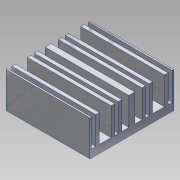
# Autodesk Inventor part: HeatSink
Saved by Autodesk Inventor 2015 (Build 190159000, 159)
## iProperties
Created: 2015-05-21
Part Number: HeatSink
Material: Aluminum 6061
Document SubType Name: Modeling
Designer: Joe Sheldon
Density: 2.7 g/cm^3
Appearance: Aluminum - Flat
Author: Joe Sheldon
Autodesk Inventor part; units mm, degrees
ref_plane "YZ Plane" through (0, 0, 0) normal (1, 0, 0) x (0, 1, 0)
ref_plane "XZ Plane" through (0, 0, 0) normal (0, 1, 0) x (-1, 0, 0)
ref_plane "XY Plane" through (0, 0, 0) normal (0, 0, 1) x (1, 0, 0)
sketch "Sketch1" plane through (0, 0, 0) normal (0, 1, 0) x (-1, 0, 0)
  line L0 (0, 0) -> (-90, 0)
  line L1 (-90, 0) -> (-90, -90)
  line L2 (-90, -90) -> (0, -90)
  line L3 (0, -90) -> (0, 0)
  dimension "d0" = 90
  dimension "d1" = 90
  constraints: 8 end point, 2 parallel, 1 horizontal, 1 perpendicular
  measures "d0" distance of L2.end L1.end
  measures "d1" distance of L1.end L0.end
extrude "Extrusion1" add sketch "Sketch1" along normal blind 88.9
sketch "Sketch2" plane through (90, 0, 0) normal (1, 0, 0) x (0, 0, -1)
  line L0 (0, 0) -> (90, 0) projected
  line L1 (90, 0) -> (90, 88.9) projected
  line L2 (0, 88.9) -> (90, 88.9) projected
  line L3 (0, 0) -> (0, 88.9) projected
  line L4 (0, 88.9) -> (1.6, 88.9)
  line L5 (0, 88.9) -> (90, 88.9) projected
  line L6 (1.6, 88.9) -> (6.2, 88.9)
  line L7 (6.2, 88.9) -> (7.8, 88.9)
  line L8 (7.8, 88.9) -> (7.8, 8.402)
  line L9 (6.2, 88.9) -> (6.2, 8.402)
  line L10 (1.6, 88.9) -> (1.6, 8.402)
  line L11 (1.6, 8.402) -> (6.2, 8.402)
  line L12 (90, 88.9) -> (88.4, 88.9)
  line L13 (88.4, 88.9) -> (88.4, 8.402)
  line L14 (88.4, 8.402) -> (83.8, 8.402)
  line L15 (83.8, 8.402) -> (83.8, 88.9)
  dimension "d4" = 1.6
  dimension "d5" = 4.6
  dimension "d6" = 1.6
  dimension "d7" = 1.6
  dimension "d8" = 4.6
  constraints: 22 end point, 5 perpendicular, 5 point on line, 2 vertical
  measures "d4" distance of L2.start L4.end
  measures "d5" distance of L4.end L6.end
  measures "d6" distance of L6.end L7.end
  measures "d7" distance of L1.end L12.end
  measures "d8" distance of L13.end L14.end
extrude "Extrusion2" cut sketch "Sketch2" against normal blind 127 contours L2 L9 L11 L10 | L13 L14 L15 L2
sketch "Sketch3" plane through (90, 0, 0) normal (1, 0, 0) x (0, 0, -1)
  line L0 (1.6, 8.402) -> (1.6, 88.9) projected
  line L1 (0, 88.9) -> (1.6, 88.9) projected
  line L2 (0, 0) -> (0, 88.9) projected
  line L3 (0, 0) -> (90, 0) projected
  line L4 (90, 0) -> (90, 88.9) projected
  line L5 (88.4, 88.9) -> (90, 88.9) projected
  line L6 (88.4, 88.9) -> (88.4, 8.402) projected
  line L7 (88.4, 8.402) -> (83.8, 8.402) projected
  line L8 (83.8, 8.402) -> (83.8, 88.9) projected
  line L9 (6.2, 88.9) -> (83.8, 88.9) projected
  line L10 (6.2, 88.9) -> (6.2, 8.402) projected
  line L11 (6.2, 8.402) -> (1.6, 8.402) projected
sketch "Sketch5" plane through (90, 0, 0) normal (1, 0, 0) x (0, 0, -1)
  line L0 (-0.0003, 88.9) -> (90, 88.9)
  line L1 (90, 88.9) -> (90, 38.1)
  line L2 (90, 38.1) -> (-0.0003, 38.1)
  line L3 (-0.0003, 38.1) -> (-0.0003, 88.9)
  point P0 (0, 0)
  dimension "d24" = 50.8
  constraints: 8 end point, 2 parallel, 1 horizontal, 1 perpendicular
  measures "d24" distance of L0.end L1.end
extrude "Extrusion3" cut sketch "Sketch5" against normal blind 111.125
sketch "Sketch6" plane through (90, 0, 0) normal (1, 0, 0) x (0, 0, -1)
  line L0 (1.6, 38.1) -> (0, 38.1) projected
  line L1 (0, 0) -> (0, 38.1) projected
  line L2 (0, 0) -> (90, 0) projected
  line L3 (90, 0) -> (90, 38.1) projected
  line L4 (90, 38.1) -> (88.4, 38.1) projected
  line L5 (88.4, 38.1) -> (88.4, 8.402) projected
  line L6 (88.4, 8.402) -> (83.8, 8.402) projected
  line L7 (83.8, 8.402) -> (83.8, 38.1) projected
  line L8 (83.8, 38.1) -> (6.2, 38.1) projected
  line L9 (6.2, 38.1) -> (6.2, 8.402) projected
  line L10 (6.2, 8.402) -> (1.6, 8.402) projected
  line L11 (1.6, 8.402) -> (1.6, 38.1) projected
  line L12 (6.2, 38.1) -> (6.2, 8.402)
  line L13 (6.2, 8.402) -> (10.01, 8.402)
  line L14 (10.01, 8.402) -> (10.01, 38.1)
  line L15 (10.01, 38.1) -> (6.2, 38.1)
  line L16 (10.01, 38.1) -> (10.01, 8.402)
  line L17 (10.01, 8.402) -> (22.71, 8.402)
  line L18 (22.71, 8.402) -> (22.71, 38.1)
  line L19 (22.71, 38.1) -> (10.01, 38.1)
  line L20 (22.71, 38.1) -> (22.71, 8.402)
  line L21 (22.71, 8.402) -> (26.52, 8.402)
  line L22 (26.52, 8.402) -> (26.52, 38.1)
  line L23 (26.52, 38.1) -> (22.71, 38.1)
  line L24 (26.52, 38.1) -> (26.52, 8.402)
  line L25 (26.52, 8.402) -> (30.33, 8.402)
  line L26 (30.33, 8.402) -> (30.33, 38.1)
  line L27 (30.33, 38.1) -> (26.52, 38.1)
  line L28 (30.33, 38.1) -> (30.33, 8.402)
  line L29 (30.33, 8.402) -> (34.14, 8.402)
  line L30 (34.14, 8.402) -> (34.14, 38.1)
  line L31 (34.14, 38.1) -> (30.33, 38.1)
  line L32 (83.8, 38.1) -> (83.8, 8.402)
  line L33 (83.8, 8.402) -> (79.99, 8.402)
  line L34 (79.99, 8.402) -> (79.99, 38.1)
  line L35 (79.99, 38.1) -> (83.8, 38.1)
  line L36 (79.99, 38.1) -> (79.99, 8.402)
  line L37 (79.99, 8.402) -> (67.29, 8.402)
  line L38 (67.29, 8.402) -> (67.29, 38.1)
  line L39 (67.29, 38.1) -> (79.99, 38.1)
  line L40 (67.29, 38.1) -> (67.29, 8.402)
  line L41 (67.29, 8.402) -> (63.48, 8.402)
  line L42 (63.48, 8.402) -> (63.48, 38.1)
  line L43 (63.48, 38.1) -> (67.29, 38.1)
  line L44 (63.48, 38.1) -> (63.48, 8.402)
  line L45 (63.48, 8.402) -> (59.67, 8.402)
  line L46 (59.67, 8.402) -> (59.67, 38.1)
  line L47 (59.67, 38.1) -> (63.48, 38.1)
  line L48 (59.67, 38.1) -> (59.67, 8.402)
  line L49 (59.67, 8.402) -> (55.86, 8.402)
  line L50 (55.86, 8.402) -> (55.86, 38.1)
  line L51 (55.86, 38.1) -> (59.67, 38.1)
  line L52 (55.86, 38.1) -> (55.86, 8.402)
  line L53 (55.86, 8.402) -> (48.24, 8.402)
  line L54 (48.24, 8.402) -> (48.24, 38.1)
  line L55 (48.24, 38.1) -> (55.86, 38.1)
  line L56 (34.14, 38.1) -> (34.14, 8.402)
  line L57 (34.14, 8.402) -> (41.76, 8.402)
  line L58 (41.76, 8.402) -> (41.76, 38.1)
  line L59 (41.76, 38.1) -> (34.14, 38.1)
  dimension "d27" = 3.81
  dimension "d28" = 12.7
  dimension "d29" = 3.81
  dimension "d30" = 3.81
  dimension "d31" = 3.81
  dimension "d32" = 3.81
  dimension "d33" = 12.7
  dimension "d34" = 3.81
  dimension "d35" = 3.81
  dimension "d36" = 3.81
  dimension "d37" = 7.62
  dimension "d38" = 7.62
  constraints: 96 end point, 27 equal length, 20 perpendicular, 1 vertical
  measures "d27" distance of L13.end L9.end
  measures "d28" distance of L17.end L13.end
  measures "d29" distance of L21.end L17.end
  measures "d30" distance of L25.end L21.end
  measures "d31" distance of L29.end L25.end
  measures "d32" distance of L6.end L33.end
  measures "d33" distance of L33.end L37.end
  measures "d34" distance of L37.end L41.end
  measures "d35" distance of L41.end L45.end
  measures "d36" distance of L45.end L49.end
  measures "d37" distance of L49.end L53.end
  measures "d38" distance of L57.end L29.end
extrude "Extrusion4" cut sketch "Sketch6" against normal blind 111.125 contours L14 L8 L18 L17 | L22 L8 L26 L25 | L30 L8 L58 L57 | L37 L38 L8 L34 | L45 L46 L8 L42 | L8 L50 L53 L54
body "Solid1"
